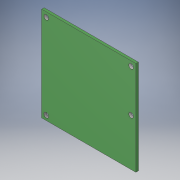
# Autodesk Inventor part: forcefoot_pcb
Saved by Autodesk Inventor 2018 (Build 220112000, 112)
## iProperties
Created: 2018-12-04
Part Number: forcefoot_pcb
Material: Generic
Document SubType Name: Modeling
Designer: jaspe
Density: 1 g/cm^3
Appearance: Default
Author: jaspe
Autodesk Inventor part; units mm, degrees
ref_plane "YZ Plane" through (0, 0, 0) normal (1, 0, 0) x (0, 1, 0)
ref_plane "XZ Plane" through (0, 0, 0) normal (0, 1, 0) x (-1, 0, 0)
ref_plane "XY Plane" through (0, 0, 0) normal (0, 0, 1) x (1, 0, 0)
sketch "Sketch1" plane through (0, 0, 0) normal (0, 1, 0) x (-1, 0, 0)
  line L0 (0, 0) -> (60, 0)
  line L1 (60, 0) -> (60, -60)
  line L2 (60, -60) -> (0, -60)
  line L3 (0, -60) -> (0, 0)
  dimension "d0" = 60
  dimension "d1" = 60
  constraints: 8 end point, 2 parallel, 1 horizontal, 1 perpendicular
  measures "d0" distance of L1.end L2.end
  measures "d1" distance of L0.end L1.end
extrude "Extrusion1" add sketch "Sketch1" along normal blind 1.6
sketch "Sketch2" plane through (0, 1.6, 0) normal (0, 1, 0) x (1, 0, 0)
  line L0 (0, 0) -> (0, 3)
  line L1 (0, 0) -> (3, 0) construction
  line L2 (0, 3) -> (-3, 3)
  line L3 (-3, 3) -> (-57, 3)
  line L4 (-3, 3) -> (51, 3) construction
  line L5 (-57, 3) -> (-57, 57)
  line L6 (-3, 3) -> (-3, 30)
  line L7 (-3, 3) -> (24, 3) construction
  circle A0 centre (-3, 30) radius 1.5
  circle A1 centre (-3, 3) radius 1.5
  circle A2 centre (-57, 3) radius 1.5
  circle A3 centre (-57, 57) radius 1.5
  dimension "d4" = 3
  dimension "d5" = 90
  dimension "d6" = 3
  dimension "d7" = 54
  dimension "d8" = 180
  dimension "d9" = 54
  dimension "d10" = 90
  dimension "d11" = 27
  dimension "d12" = 90
  dimension "d13" = 3
  dimension "d14" = 3
  dimension "d15" = 3
  dimension "d16" = 3
  constraints: 16 end point, 4 centre point, 4 coincident, 4 horizontal, 3 equal length, 2 perpendicular, 2 vertical
  measures "d4" distance of L0.start L0.end
  measures "d5" angle of L1 L0
  measures "d6" distance of L0.end L2.end
  measures "d7" distance of L2.end L3.end
  measures "d8" angle of L3 L4
  measures "d9" distance of L3.end L5.end
  measures "d10" angle of L3 L5
  measures "d11" distance of L2.end L6.end
  measures "d12" angle of L7 L6
  measures "d13" diameter of A0
  measures "d14" diameter of A1
  measures "d15" diameter of A2
  measures "d16" diameter of A3
extrude "Extrusion2" cut sketch "Sketch2" against normal up to surface (1.6 mm away)
body "Solid1"
